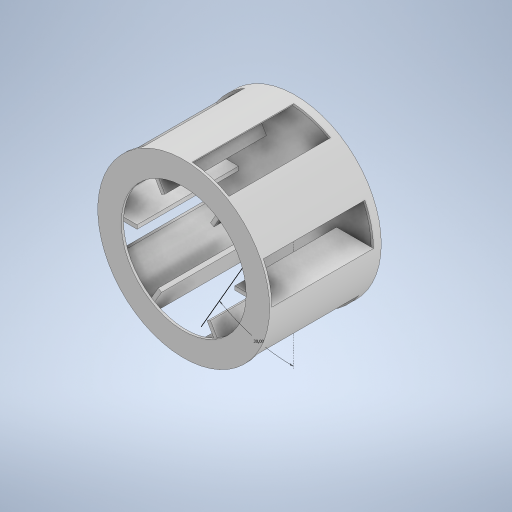
# Autodesk Inventor part: Cilindro do Motor Industrial
Saved by Autodesk Inventor 2023 (Build 270158030, 158C)
## iProperties
Created: 2022-07-18
Part Number: Cilindro do Motor Industrial
Material: Generic
Document SubType Name: Modeling
Designer: coqui
Density: 1 g/cm^3
Appearance: Default
Author: coqui
Autodesk Inventor part; units mm, degrees
ref_plane "YZ Plane" through (0, 0, 0) normal (1, 0, 0) x (0, 1, 0)
ref_plane "XZ Plane" through (0, 0, 0) normal (0, 1, 0) x (-1, 0, 0)
ref_plane "XY Plane" through (0, 0, 0) normal (0, 0, 1) x (1, 0, 0)
sketch "Sketch1" plane through (0, 0, 0) normal (0, 0, 1) x (1, 0, 0)
  circle A0 centre (0, 0) radius 55
  dimension "d0" = 110
  constraints: 1 centre point, 1 coincident
  measures "d0" diameter of A0
extrude "Extrusion1" add sketch "Sketch1" along normal blind 71.5
shell "Shell1" thickness 1.5 removed faces 1 at (13.749, -10.4033, 71.5)
sketch "Sketch2" plane through (0, 0, 71.5) normal (0, 0, 1) x (1, 0, 0)
  circle A0 centre (0, 0) radius 55 projected
  circle A1 centre (0, 0) radius 55
  circle A2 centre (0, 0) radius 40
  dimension "d4" = 110
  dimension "d5" = 80
  constraints: 2 centre point, 2 coincident
  measures "d4" diameter of A1
  measures "d5" diameter of A2
extrude "Extrusion2" add sketch "Sketch2" against normal blind 1.5
sketch "Sketch3" plane through (0, 0, 0) normal (0, 0, -1) x (-1, 0, 0)
  circle A0 centre (0, 0) radius 15
  dimension "d8" = 30
  constraints: 1 centre point, 1 coincident
  measures "d8" diameter of A0
extrude "Extrusion3" add sketch "Sketch3" along normal blind 25
sketch "Sketch4" plane through (0, 0, -25) normal (0, 0, -1) x (-1, 0, 0)
  circle A0 centre (0, 0) radius 7.5
  dimension "d11" = 15
  constraints: 1 centre point, 1 coincident
  measures "d11" diameter of A0
extrude "Extrusion4" cut sketch "Sketch4" against normal blind 25
sketch "Sketch5" plane through (0, 0, 1.5) normal (0, 0, 1) x (1, 0, 0)
  circle A0 centre (0, 0) radius 7.5 construction
  line L0 (0, 0) -> (0, -95.8386) construction
  line L1 (0, 0) -> (-58.9042, -102.025)
  dimension "d14" = 30
  constraints: 4 end point, 1 vertical
  measures "d14" angle of L1 L0
ref_plane "Work Plane1" through (-58.9042, -102.025, 1.5) normal (-0.5, -0.8660254, 0) x (0.8660254, -0.5, 0)
sketch "Sketch7" plane through (-58.9042, -102.025, 1.5) normal (-0.5, -0.8660254, 0) x (0.8660254, -0.5, 0)
  line L0 (53.5, 0) -> (-53.5, 0) projected
  line L1 (55, -1.5) -> (-55, -1.5) projected
  line L2 (0, 3.5) -> (24, 3.5)
  line L3 (24, 3.5) -> (24, 68.5)
  line L4 (24, 68.5) -> (0, 68.5)
  line L5 (0, 68.5) -> (0, 3.5)
  line L6 (55, 70) -> (-55, 70) projected
  point P0 (0, -1.5)
  point P1 (0, -1.5)
  dimension "d18" = 5
  dimension "d19" = 65
  dimension "d20" = 24
  dimension "d21" = 0
  dimension "d22" = 1.5
  constraints: 8 end point, 2 parallel, 1 horizontal, 1 midpoint, 1 perpendicular
  measures "d18" distance between parallel lines of L1 L2
  measures "d19" distance of L2.end L3.end
  measures "d20" distance of L3.end L4.end
  measures "d21" distance from line of point (0, -1.5) L5
  measures "d22" distance between parallel lines of L4 L6
extrude "Extrusion5" cut sketch "Sketch7" against normal blind 110.75
pattern_circular "Circular Pattern1" count 6 over 360 about axis through (0, 0, 0) along (0, 0, 1) of "Extrusion5"
sketch "Sketch12" plane through (0, 0, 5) normal (0, 0, 1) x (0.9579572, -0.286911, 0)
  line L0 (9.6549, 29.9119) -> (14.7648, 51.483)
  line L1 (14.7648, 51.483) -> (14.9013, 52.0593)
  line L2 (7.2222, 30.4881) -> (12.3321, 52.0593)
  line L3 (12.3321, 52.0593) -> (12.4686, 52.6356)
  line L4 (14.9013, 52.0593) -> (12.4686, 52.6356)
  line L5 (12.6779, 53.5189) -> (12.3321, 52.0593) projected
  line L6 (9.6549, 29.9119) -> (7.2222, 30.4881)
  point P0 (0, 0)
  point P1 (8.4385, 30.2)
  dimension "d34" = 2.5
  dimension "d35" = 30.2
  constraints: 12 end point, 2 collinear, 2 perpendicular, 1 midpoint, 1 point on line
  measures "d34" distance between parallel lines of L0 L2
  measures "d35" vertical distance of point (0, 0) point (8.439, 30.2)
extrude "Extrusion7" add sketch "Sketch12" along normal blind 65
pattern_circular "Circular Pattern2" count 6 over 360 about axis through (0, 0, -25) along (0, 0, 1) of "Extrusion7"
body "Solid1"
